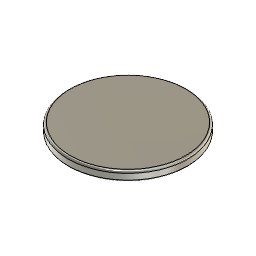
Load Platform (Autodesk Fusion 360 design; units mm, degrees)
Autodesk Fusion 360 part; units mm, degrees
cylinder "CylinderPrimitive1" add diameter 60 height 5 placed x (1, 0, 0) y (0, 1, 0) z (0, 0, 1) at (0, 0, 0)
fillet "Fillet1" radius 1 2 edges at (-27.9698, -10.8485, 5) (-27.9698, 10.8485, 0)
